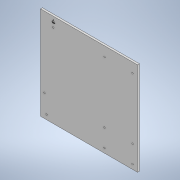
# Autodesk Inventor part: MotherboardBase
Saved by Autodesk Inventor 2020 (Build 240168000, 168)
## iProperties
Created: 2026-07-11
Part Number: MotherboardBase
Material: Generic
Document SubType Name: Modeling
Designer: Nessa
Density: 1 g/cm^3
Appearance: Default
Author: Nessa
Autodesk Inventor part; units mm, degrees
ref_plane "YZ Plane" through (0, 0, 0) normal (1, 0, 0) x (0, 1, 0)
ref_plane "XZ Plane" through (0, 0, 0) normal (0, 1, 0) x (-1, 0, 0)
ref_plane "XY Plane" through (0, 0, 0) normal (0, 0, 1) x (1, 0, 0)
sketch "Sketch1" plane through (0, 0, 0) normal (0, 0, 1) x (1, 0, 0)
  line L0 (-125, 120) -> (125, 120)
  line L1 (125, 120) -> (125, -120)
  line L2 (125, -120) -> (-125, -120)
  line L3 (-125, -120) -> (-125, 120)
  point P0 (0, 0)
  dimension "d0" = 250
  dimension "d1" = 240
  dimension "d2" = 125
  dimension "d3" = 120
  constraints: 8 end point, 2 parallel, 1 horizontal, 1 perpendicular
  measures "d0" distance of L1.end L2.end
  measures "d1" distance of L0.end L1.end
  measures "d2" distance from line of L3 point (0, 0)
  measures "d3" distance from line of L0 point (0, 0)
extrude "Extrusion1" add sketch "Sketch1" along normal mid plane 5
sketch "Sketch3" plane through (0, 0, 2.5) normal (0, 0, 1) x (1, 0, 0)
  line L0 (125, 120) -> (-125, 120) projected
  line L1 (-115, 95) -> (-115, -108.2)
  line L2 (-125, -120) -> (125, -120) projected
  line L3 (-92.14, 95) -> (-92.14, -120)
  line L4 (39.94, 95) -> (39.94, -108.2)
  line L5 (112.33, 95) -> (112.33, -108.2)
  line L6 (125, -120) -> (125, 120)
  line L7 (112.33, -62.48) -> (-115, -62.48)
  line L8 (-125, 120) -> (-125, -120)
  line L9 (112.33, -108.2) -> (-115, -108.2)
  line L10 (-115, 95) -> (112.33, 95)
  point P0 (0, 0)
  point P1 (-109.3528, -107.8905)
  point P2 (39.9365, -62.4666)
  dimension "d6" = 10
  dimension "d7" = 22.86
  dimension "d8" = 132.08
  dimension "d9" = 72.39
  dimension "d11" = 25
  dimension "d12" = 157.48
  dimension "d13" = 45.72
  constraints: 22 end point, 6 perpendicular, 5 point on line
  measures "d6" distance between parallel lines of L8 L1
  measures "d7" distance between parallel lines of L3 L1
  measures "d8" distance between parallel lines of L4 L3
  measures "d9" distance between parallel lines of L5 L4
  measures "d11" distance between parallel lines of L0 L10
  measures "d12" distance between parallel lines of L7 L10
  measures "d13" distance between parallel lines of L7 L9
hole "Hole1" at (-92.14, 95, 2.5) at (39.94, 95, 2.5) at (112.33, 95, 2.5) at (112.33, -62.48, 2.5) at (112.33, -108.2, 2.5) at (39.94, -108.2, 2.5) at (-109.3528, -107.8905, 2.5) at (-115, -62.48, 2.5) at (39.9365, -62.4666, 2.5) direction (0, 0, -1) diameter 3.6 end through all
sketch "Sketch4" plane through (0, 0, 2.5) normal (0, 0, 1) x (1, 0, 0)
  line L0 (-92.14, 112.7708) -> (-92.14, 107.7708)
  line L1 (-92.14, 107.7708) -> (-89.64, 107.7708)
  line L2 (-89.64, 107.7708) -> (-92.14, 112.7708)
  circle A0 centre (-92.14, 95) radius 1.8 projected
  line L3 (-92.14, 107.7708) -> (-94.64, 107.7708)
  line L4 (-94.64, 107.7708) -> (-92.14, 112.7708)
  line L5 (-96.2888, 106.9952) -> (-87.7345, 106.9952) construction
  line L6 (-87.7345, 106.9952) -> (-87.7345, 103.8167) construction
  line L7 (-87.7345, 103.8167) -> (-96.2888, 103.8167) construction
  line L8 (-96.2888, 103.8167) -> (-96.2888, 106.9952) construction
  line L9 (-95.3867, 103.8809) -> (-95.3867, 106.3501)
  line L10 (-95.3867, 106.3501) -> (-96.2888, 106.3501)
  line L11 (-96.2888, 106.3501) -> (-96.2888, 106.9309)
  line L12 (-96.2888, 106.9309) -> (-93.7183, 106.9309)
  line L13 (-93.7183, 106.9309) -> (-93.7183, 106.3501)
  line L14 (-93.7183, 106.3501) -> (-94.6205, 106.3501)
  line L15 (-94.6205, 106.3501) -> (-94.6205, 103.8809)
  line L16 (-94.6205, 103.8809) -> (-95.3867, 103.8809)
  spline S0 degree 2 poles (-90.6288, 105.4059) (-90.6288, 104.6645) (-91.4197, 103.8167) (-92.1068, 103.8167) knots 0 0 0 1 2 2 2
  spline S1 degree 2 poles (-92.1068, 103.8167) (-92.7964, 103.8167) (-93.5824, 104.6743) (-93.5824, 105.4059) knots 0 0 0 1 2 2 2
  spline S2 degree 2 poles (-93.5824, 105.4059) (-93.5824, 106.14) (-92.7964, 106.9952) (-92.1068, 106.9952) knots 0 0 0 1 2 2 2
  spline S3 degree 2 poles (-92.1068, 106.9952) (-91.4197, 106.9952) (-90.6288, 106.145) (-90.6288, 105.4059) knots 0 0 0 1 2 2 2
  spline S4 degree 2 poles (-91.4197, 105.4059) (-91.4197, 105.6803) (-91.5309, 106.0634) (-91.6273, 106.1845) knots 0 0 0 1 2 2 2
  spline S5 degree 2 poles (-91.6273, 106.1845) (-91.7237, 106.3106) (-91.9709, 106.4193) (-92.1043, 106.4193) knots 0 0 0 1 2 2 2
  spline S6 degree 2 poles (-92.1043, 106.4193) (-92.2452, 106.4193) (-92.4751, 106.318) (-92.5813, 106.1895) knots 0 0 0 1 2 2 2
  spline S7 degree 2 poles (-92.5813, 106.1895) (-92.6753, 106.0708) (-92.7914, 105.6778) (-92.7914, 105.4059) knots 0 0 0 1 2 2 2
  spline S8 degree 2 poles (-92.7914, 105.4059) (-92.7914, 105.1242) (-92.6802, 104.7534) (-92.5838, 104.6274) knots 0 0 0 1 2 2 2
  spline S9 degree 2 poles (-92.5838, 104.6274) (-92.4874, 104.5013) (-92.2378, 104.3926) (-92.1043, 104.3926) knots 0 0 0 1 2 2 2
  spline S10 degree 2 poles (-92.1043, 104.3926) (-91.9684, 104.3926) (-91.7163, 104.5087) (-91.6248, 104.6323) knots 0 0 0 1 2 2 2
  spline S11 degree 2 poles (-91.6248, 104.6323) (-91.526, 104.7658) (-91.4197, 105.1192) (-91.4197, 105.4059) knots 0 0 0 1 2 2 2
  spline S12 degree 2 poles (-87.8284, 105.9695) (-87.8284, 105.7569) (-87.9643, 105.3713) (-88.0904, 105.2428) knots 0 0 0 1 2 2 2
  spline S13 degree 2 poles (-88.0904, 105.2428) (-88.167, 105.1613) (-88.3549, 105.0278) (-88.4661, 104.9808) knots 0 0 0 1 2 2 2
  spline S14 degree 2 poles (-88.4661, 104.9808) (-88.5798, 104.9339) (-88.8442, 104.8795) (-89.0074, 104.8795) knots 0 0 0 1 2 2 2
  line L17 (-89.0074, 104.8795) -> (-89.4078, 104.8795)
  line L18 (-89.4078, 104.8795) -> (-89.4078, 103.8809)
  line L19 (-89.4078, 103.8809) -> (-90.174, 103.8809)
  line L20 (-90.174, 103.8809) -> (-90.174, 106.9309)
  line L21 (-90.174, 106.9309) -> (-88.9901, 106.9309)
  spline S15 degree 2 poles (-88.9901, 106.9309) (-88.7281, 106.9309) (-88.345, 106.8346) (-88.1893, 106.7307) knots 0 0 0 1 2 2 2
  spline S16 degree 2 poles (-88.1893, 106.7307) (-88.0162, 106.6146) (-87.8284, 106.2339) (-87.8284, 105.9695) knots 0 0 0 1 2 2 2
  spline S17 degree 2 poles (-88.6144, 105.9497) (-88.6144, 106.0807) (-88.738, 106.2661) (-88.822, 106.3007) knots 0 0 0 1 2 2 2
  spline S18 degree 2 poles (-88.822, 106.3007) (-88.9307, 106.3476) (-89.1285, 106.3625) (-89.299, 106.3625) knots 0 0 0 1 2 2 2
  line L22 (-89.299, 106.3625) -> (-89.4078, 106.3625)
  line L23 (-89.4078, 106.3625) -> (-89.4078, 105.448)
  line L24 (-89.4078, 105.448) -> (-89.3534, 105.448)
  spline S19 degree 2 poles (-89.3534, 105.448) (-89.2471, 105.448) (-89.0543, 105.4529) (-88.9826, 105.4653) knots 0 0 0 1 2 2 2
  spline S20 degree 2 poles (-88.9826, 105.4653) (-88.9209, 105.4752) (-88.7849, 105.5345) (-88.7478, 105.5715) knots 0 0 0 1 2 2 2
  spline S21 degree 2 poles (-88.7478, 105.5715) (-88.6687, 105.6457) (-88.6144, 105.8113) (-88.6144, 105.9497) knots 0 0 0 1 2 2 2
  point P0 (0, 0)
  dimension "d21" = 5
  constraints: 10 end point, 1 perpendicular, 1 symmetric about line, 1 vertical, 2 other
  measures "d21" distance of L0.start L0.end
extrude "Extrusion2" cut sketch "Sketch4" against normal blind 2.5 contours L2 L1 L0 | L0 L3 L4 | L9 L10 L11 L12 L13 L14 L15 L16 | S0 S1 S2 S3 | S12 S13 S14 L17 L18 L19 L20 L21 S15 S16
equation "\"d2\" = 0.5 * d0"
equation "\"d3\" = 0.5 * d1"
body "Solid1"
